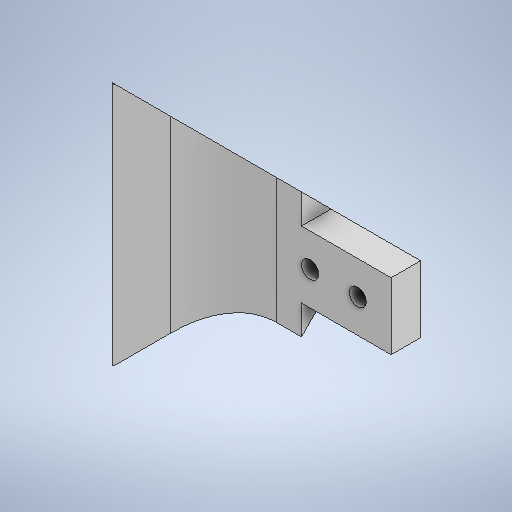
# Autodesk Inventor part: KickerFoot
Saved by Autodesk Inventor 2025.1 (Build 291241000, 241)
## iProperties
Created: 2026-04-18
Part Number: KickerFoot
Material: Generic
Document SubType Name: Modeling
Designer: User
Density: 1 g/cm^3
Appearance: Default
Author: User
## iProperties of the stored document KickerFoot_3DPrint.ipt
Created: 2026-04-18
Part Number: KickerFoot_3DPrint
Material: Generic
Document SubType Name: Modeling
Designer: User
Density: 1 g/cm^3
Appearance: Default
Author: User
Autodesk Inventor part; units mm, degrees
ref_plane "YZ Plane" through (0, 0, 0) normal (1, 0, 0) x (0, 1, 0)
ref_plane "XZ Plane" through (0, 0, 0) normal (0, 1, 0) x (-1, 0, 0)
sketch "Sketch1" plane through (0, 0, 0) normal (0, 0, 1) x (1, 0, 0)
  circle A0 centre (-4.0482, 0) radius 1.45 projected
  circle A1 centre (4.0482, 0) radius 1.45 projected
  line L0 (-8, 3.9518) -> (-8, -3.9518) projected
  line L1 (-8, -3.9518) -> (8, -3.9518) projected
  line L2 (8, -3.9518) -> (8, 3.9518) projected
  line L3 (8, 3.9518) -> (-8, 3.9518) projected
  line L4 (8.2, 4.1518) -> (8.2, -4.1518)
  line L5 (8.2, -4.1518) -> (-8.2, -4.1518)
  line L6 (-8.2, -4.1518) -> (-8.2, 4.1518)
  line L7 (-8.2, 4.1518) -> (8.2, 4.1518)
  point P0 (0, 0)
  dimension "d0" = 0.2
  constraints: 8 end point, 3 other
  measures "d0" distance between parallel lines of L2 L4
extrude "Extrusion1" add sketch "Sketch1" along normal blind 2 contours L3 L2 L1 L0 | L4 L5 L6 L7
sketch "Sketch2" plane through (0, 0, 2) normal (0, 0, 1) x (1, 0, 0)
  line L0 (8.2, -4.1518) -> (8.2, 4.1518) projected
  line L1 (8.2, 4.1518) -> (-8.2, 4.1518) projected
  line L2 (-8.2, 4.1518) -> (-8.2, -4.1518) projected
  line L3 (-8.2, -4.1518) -> (8.2, -4.1518) projected
  line L4 (9.7, 5.6518) -> (9.7, -5.6518)
  line L5 (9.7, -5.6518) -> (-9.7, -5.6518)
  line L6 (-9.7, -5.6518) -> (-9.7, 5.6518)
  line L7 (-9.7, 5.6518) -> (9.7, 5.6518)
  point P0 (0, 0)
  dimension "d3" = 1.5
  constraints: 8 end point, 3 other
  measures "d3" distance between parallel lines of L0 L4
ref_plane "Work Plane1" through (7.9977, -5.9583, -3) normal (0, 0, 1) x (1, 0, 0)
extrude "Extrusion2" add sketch "Sketch2" against normal up to surface (5 mm away)
sketch "Sketch3" plane through (-9.7, 5.6518, 2) normal (0, 1, 0) x (1, 0, 0)
  line L0 (0, 0) -> (0, 5) projected
  line L1 (0, 0) -> (0, -18)
  circle A0 centre (0, -18) radius 18
  circle A1 centre (0, -18) radius 23
  line L2 (0, -18) -> (-16.2635, -1.7365)
  line L3 (0, -18) -> (23, -18) construction
  point P0 (9.7, 2)
  point P1 (-12.7279, -5.2721)
  dimension "d6" = 18
  dimension "d7" = 135
  constraints: 6 end point, 2 coincident, 2 point on circle, 1 centre point, 1 equal length, 1 horizontal, 1 vertical, 3 other
  measures "d6" distance of L0.start L1.end
  measures "d7" angle of L3 L2
extrude "Extrusion3" add sketch "Sketch3" against normal up to surface (11.3036 mm away) contours A0 L2 A1 L0 picked at (-13.0139, -1.2154)
sketch "Sketch5" plane through (9.7, 5.6518, 2) normal (0, 1, 0) x (1, 0, 0)
  line L0 (-35.6635, -1.7365) -> (-32.1279, -5.2721) projected
  line L1 (-35.6635, -1.7365) -> (-32.1279, -5.2721)
  line L2 (-32.1279, -5.2721) -> (-37.0777, -10.2218)
  line L3 (-37.0777, -10.2218) -> (-40.6132, -6.6863)
  line L4 (-40.6132, -6.6863) -> (-35.6635, -1.7365)
  point P0 (-9.7, 2)
  dimension "d10" = 7
  constraints: 8 end point, 3 equal length, 1 perpendicular
  measures "d10" distance of L0.end L2.end
extrude "Extrusion4" add sketch "Sketch5" against normal up to surface (11.3036 mm away)
sketch "Sketch6" plane through (9.7, -5.6518, -3) normal (0, -1, 0) x (1, 0, 0)
  line L0 (-37.0777, 15.2218) -> (-32.1279, 10.2721) projected
  arc A0 (-32.1279, 10.2721) -> (-19.4, 5) centre (-19.4, 23) ccw projected
  line L1 (-40.6132, 11.6863) -> (-37.0777, 15.2218) projected
  line L2 (-35.6635, 6.7365) -> (-40.6132, 11.6863) projected
  arc A1 (-35.6635, 6.7365) -> (-19.4, 0) centre (-19.4, 23) ccw projected
  line L3 (-19.4, 5) -> (0, 5) projected
  line L4 (0, 0) -> (-19.4, 0) projected
  line L5 (-15.1982, 5) -> (-15.1982, 3) projected
  line L6 (-15.1982, 5) -> (-15.1982, 0)
  point P0 (-9.7, 3)
  constraints: 3 point on line, 2 end point, 1 perpendicular
extrude "Extrusion5" add sketch "Sketch6" along normal blind 15
sketch "Sketch7" plane through (9.7, 5.6518, 2) normal (0, 1, 0) x (1, 0, 0)
  line L0 (-32.1279, -5.2721) -> (-37.0777, -10.2218) projected
  line L1 (-37.0777, -10.2218) -> (-40.6132, -6.6863) projected
  line L2 (-40.6132, -6.6863) -> (-35.6635, -1.7365) projected
  arc A0 (-19.4, 5) -> (-35.6635, -1.7365) centre (-19.4, -18) ccw projected
  line L3 (-19.4, 5) -> (-15.1982, 5) projected
  line L4 (-15.1982, 5) -> (-15.1982, 0) projected
  line L5 (-15.1982, 0) -> (-19.4, 0) projected
  arc A1 (-19.4, 0) -> (-32.1279, -5.2721) centre (-19.4, -18) ccw projected
  point P0 (-9.7, 2)
extrude "Extrusion6" add sketch "Sketch7" along normal blind 15
sketch "Sketch8" plane through (-5.4982, 5.6518, 2) normal (1, 0, 0) x (0, 0, -1)
  line L0 (-43.306, 51.1457) -> (8.0398, -0.2) projected
  line L1 (8.0154, -11.1036) -> (-43.306, -62.425) projected
  line L2 (-44.7202, 49.7315) -> (6.6255, -1.6142)
  line L3 (6.6012, -9.6894) -> (-44.7202, -61.0108)
  line L4 (5, 0) -> (5, 15) projected
  line L5 (-10.2218, 15) -> (-5.2721, 15) projected
  line L6 (-5.2721, 15) -> (0, 15) projected
  line L7 (0, 15) -> (5, 15) projected
  line L8 (5, -11.3036) -> (5, -26.3036) projected
  line L9 (5, -26.3036) -> (0, -26.3036) projected
  line L10 (0, -26.3036) -> (-5.2721, -26.3036) projected
  line L11 (-5.2721, -26.3036) -> (-10.2218, -26.3036) projected
  line L12 (0, -11.3036) -> (5, -11.3036) projected
  point P0 (2, -5.6518)
  point P1 (-9.9887, 15)
  point P2 (5, 0.0113)
  point P3 (4.987, -11.3036)
  point P4 (-10.013, -26.3036)
  dimension "d17" = 2
  dimension "d18" = 2
  constraints: 4 end point, 2 parallel
  measures "d17" distance between parallel lines of L0 L2
  measures "d18" distance between parallel lines of L1 L3
extrude "Extrusion7" cut sketch "Sketch8" against normal through all
body "Solid1"
